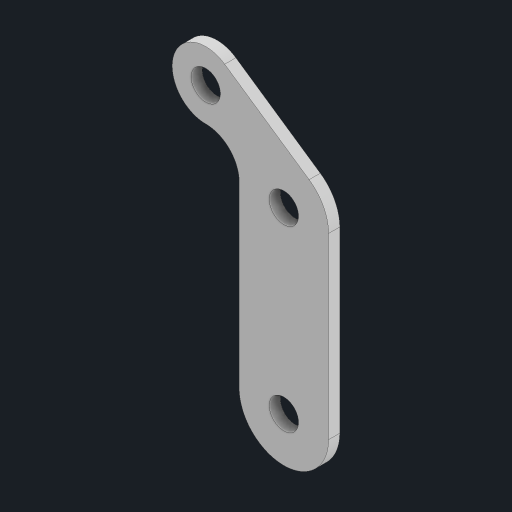
# Autodesk Inventor part: brace_gusset
Saved by Autodesk Inventor 2024 (Build 280153000, 153)
## iProperties
Created: 2023-08-16
Part Number: brace_gusset
Material: Generic
Document SubType Name: Modeling
Designer: avere
Density: 1 g/cm^3
Appearance: Default
Author: avere
Autodesk Inventor part; units mm, degrees
ref_plane "YZ Plane" through (0, 0, 0) normal (1, 0, 0) x (0, 1, 0)
ref_plane "XZ Plane" through (0, 0, 0) normal (0, 1, 0) x (-1, 0, 0)
ref_plane "XY Plane" through (0, 0, 0) normal (0, 0, 1) x (1, 0, 0)
sketch "Sketch1" plane through (0, 0, 0) normal (0, 0, 1) x (1, 0, 0)
  circle A0 centre (9.9098, 12.6224) radius 2.0828
  circle A1 centre (9.9098, -12.7776) radius 2.0828
  arc A2 (16.2598, 12.6224) -> (13.495, 17.8634) centre (9.9098, 12.6224) ccw
  arc A3 (3.5598, -12.7776) -> (16.2598, -12.7776) centre (9.9098, -12.7776) ccw
  line L0 (3.5598, 12.6224) -> (3.5598, -12.7776)
  line L1 (16.2598, 12.6224) -> (16.2598, -12.7776)
  circle A4 centre (-1.2027, 22.1474) radius 2.0828
  arc A5 (1.4862, 26.0782) -> (-1.2027, 17.3849) centre (-1.2027, 22.1474) ccw
  arc A6 (3.5598, 12.6224) -> (-1.2027, 17.3849) centre (-1.2027, 12.6224) ccw
  line L2 (1.4862, 26.0782) -> (13.495, 17.8634)
  point P0 (0, 0)
  dimension "d0" = 4.1656
  dimension "d1" = 12.7
  dimension "d2" = 9.525
  constraints: 8 point on circle, 7 centre point, 6 end point, 6 tangent, 3 coincident, 2 other
  measures "d0" diameter of A1
  measures "d1" diameter of A3
  measures "d2" diameter of A5
extrude "Extrusion1" add sketch "Sketch1" along normal blind 1.5875
body "Solid1"
